Autodesk Fusion 360 part; units mm, degrees
note: some values were not read from the file. Chosen so that the rebuilt part matches the saved one: which face or edge a step refers to; which pieces of a blend or face edit are solid. Set by a fixed rule: which sketch regions a step uses.
(part 3 of 3)
extrude "Extrude62" cut sketch "Sketch8" along normal blind 2 contours L4 L5 L6 L7 | L14 L15 L16 L18 | L24 L25 L26 L27 | L31 L32 L34 L35 | L50 L51 L52 L54 | L56 L60 L61 L62 | L67 L68 L69 L70 | L73 L74 L75 L76 picked at (-28.883331, 26.433334) picked at (-28.883331, 19.533334) picked at (-28.883331, 12.633334) picked at (-27.116664, 3.966667) picked at (-27.116664, -9.833333) picked at (-27.116664, -16.733333) picked at (-27.116664, -23.633333) picked at (-28.833331, -1.216666) bodies 14
extrude "Extrude63" add sketch "Sketch8" against normal blind 1.1 separate body contours L79 L80 L81 L83 | L85 L86 L90 L92 | L93 L94 L98 L99 | L101 L103 L106 L107 | L109 L110 L111 L115 L116 L118 L119 L120 | L121 L122 L126 L128 | L129 L130 L134 L136 | L137 L138 L141 L144 picked at (31.150002, 24.666667) picked at (28.883336, 15.5) picked at (27.116669, 14.9) picked at (31.150002, 3.966667) picked at (25.100002, -1.744392) picked at (28.883336, -12.1) picked at (27.116669, -12.7) picked at (31.150002, -21.866666) makes body 48 at (-28.883336, 48, -12.1) makes body 49 at (-28.883336, 48, 15.5) makes body 50 at (-27.116669, 48, 14.9) makes body 51 at (-27.116669, 48, -12.7) makes body 52 at (-27.116669, 48, 1.1) makes body 53 at (-31.150002, 48, 24.666667) makes body 54 at (-31.150002, 48, 3.966667) makes body 55 at (-31.150002, 48, -21.866666)
extrude "Extrude64" cut sketch "Sketch8" along normal blind 2 contours L77 L78 L82 L84 | L87 L88 L89 L91 | L95 L96 L97 L100 | L102 L104 L105 L108 | L112 L113 L114 L117 | L123 L124 L125 L127 | L131 L132 L133 L135 | L139 L140 L142 L143 picked at (27.116669, 26.433334) picked at (27.116669, 19.533334) picked at (27.116669, 12.633334) picked at (28.883336, 3.966667) picked at (27.116669, -1.166666) picked at (27.116669, -9.833333) picked at (28.883336, -16.733333) picked at (28.883336, -23.633333) bodies 14
extrude "Extrude65" add sketch "Sketch8" against normal blind 1.5 separate body contours A7 A8 L180 L182 | A7 L0 L180 L182 | A7 L166 L167 | A7 A8 L166 L167 | L0 L180 L181 L182 | A8 L179 L180 L182 | A8 L165 A47 L166 L168 L169 | A7 L170 L172 L173 | A7 A8 L170 L173 | A8 L170 L171 A48 L174 L177 L178 | A9 | A14 | A15 | A18 | A21 | A24 | A27 | A30 | A33 | A36 | A39 | L145 L146 L147 L148 L149 L150 L160 A44 A45 L161 A46 L162 L163 L164 | L151 L152 L153 L154 A42 L155 L156 L157 L158 A43 L159 L175 L176 A49 picked at (-7.789481, -16.486527) picked at (-2.132077, -15.94653) picked at (8.537855, 14.819051) picked at (11.812408, 13.909637) picked at (-2.965568, -13.564981) picked at (-4.098713, -22.481866) picked at (11.913762, 18.236099) picked at (-10.040864, 13.380579) picked at (-12.96051, 13.151425) picked at (-16.55466, 13.557623) picked at (-14.046923, 17.368666) picked at (-14.046923, 25.368666) picked at (18.953077, 25.368666) picked at (18.953077, 17.368666) picked at (40.611389, 27.41376) picked at (40.611389, -20.88624) picked at (18.953077, -22.931334) picked at (1.953077, -22.931334) picked at (-14.046923, -22.931334) picked at (-38.388611, -20.88624) picked at (-38.388611, 27.41376) picked at (39.267618, 1.119707) picked at (-40.432767, 2.078113) makes body 56 at (-11.533333, 48, 18.484122) makes body 57 at (14.814326, 48, 13.85056) makes body 58 at (-40.466668, 48, 1.116667) makes body 59 at (40.432767, 48, 2.078113) makes body 60 at (0.051541, 48, -15.525326)
move_body "Move5" bodies 56 59 57 58 60 to x (1, 0, 0) y (0, 1, 0) z (0, 0, 1) at (0, -10, 0)
move_face "OffsetFaces18" offset 7 1 faces at (24.599998, 37.5, 26.683334) on bodies 59
move_face "OffsetFaces19" offset 8 7 faces at (24.599998, 37.5, 19.783334) (24.599998, 37.5, 12.883334) (24.599998, 37.5, 5.983334) (24.599998, 37, -3.183333) (24.599998, 37.5, -7.816666) (24.599998, 37.5, -14.716666) (24.599998, 37.5, -21.616666) on bodies 59
move_face "OffsetFaces20" offset 7 8 faces at (-31.400002, 37.5, 26.683334) (-31.400002, 37.5, 19.783334) (-31.400002, 37.5, 12.883334) (-31.400002, 37.5, 5.983334) (-31.400002, 37, -3.183333) (-31.400002, 37.5, -7.816666) (-31.400002, 37.5, -14.716666) (-31.400002, 37.5, -21.616666) on bodies 58
hidden bodies 36 37 38 39 1 7 8 9 35
named bodies: "Deleted", "Screw1-1", "Screw1-2", "Screw1-3", "Screw2-1", "Screw2-2", "Screw2-3", "Screw3-1", "Screw3-2", "Screw3-3", "ScreenHolder"
